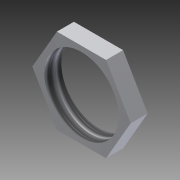
# Autodesk Inventor part: LED Holder Nut
Saved by Autodesk Inventor 2015 (Build 190159000, 159)
## iProperties
Created: 2015-11-02
Part Number: LED Holder Nut
Material: ABS Plastic
Document SubType Name: Modeling
Designer: James
Density: 1.06 g/cm^3
Appearance: Smooth - White
Author: James
Autodesk Inventor part; units mm, degrees
ref_plane "YZ Plane" through (0, 0, 0) normal (1, 0, 0) x (0, 1, 0)
ref_plane "XZ Plane" through (0, 0, 0) normal (0, 1, 0) x (-1, 0, 0)
ref_plane "XY Plane" through (0, 0, 0) normal (0, 0, 1) x (1, 0, 0)
sketch "Sketch1" plane through (0, 0, 0) normal (0, 1, 0) x (-1, 0, 0)
  circle A0 centre (0, 0) radius 4.3656
  line L0 (5.7735, 0) -> (2.8868, -5)
  line L1 (2.8868, -5) -> (-2.8868, -5)
  line L2 (-2.8868, -5) -> (-5.7735, 0)
  line L3 (-5.7735, 0) -> (-2.8868, 5)
  line L4 (-2.8868, 5) -> (2.8868, 5)
  line L5 (2.8868, 5) -> (5.7735, 0)
  dimension "d0" = 8.7312
  dimension "d1" = 10
  constraints: 12 end point, 2 coincident, 1 centre point, 13 other
  measures "d0" diameter of A0
  measures "d1" distance between parallel lines of L1 L4
extrude "Extrusion1" add sketch "Sketch1" along normal blind 2
thread "Thread1" size "M9x1.25" class "6H" standard "ANSI Metric M Profile" full length
body "Solid1"
